Autodesk Fusion 360 part; units mm, degrees
note: some values were not read from the file. Set by a fixed rule: which sketch regions a step uses.
(part 2 of 3)
  line L909 (149.682, -103.079) -> (149.715, -103.248)
  line L910 (149.715, -103.248) -> (149.715, -103.421)
  line L911 (149.715, -103.421) -> (149.682, -103.59)
  line L912 (149.682, -103.59) -> (149.616, -103.749)
  line L913 (144.253, -97.1502) -> (144.186, -96.9907)
  line L914 (144.186, -96.9907) -> (144.153, -96.8214)
  line L915 (144.153, -96.8214) -> (144.153, -96.6488)
  line L916 (129.784, -101.74) -> (129.88, -101.597)
  line L917 (129.88, -101.597) -> (130.002, -101.475)
  line L918 (144.471, -96.0544) -> (144.614, -95.9585)
  line L919 (144.614, -95.9585) -> (144.774, -95.8925)
  line L920 (138.289, -101.26) -> (138.289, -101.432)
  line L921 (138.289, -101.432) -> (138.255, -101.601)
  line L922 (144.774, -95.8925) -> (144.943, -95.8588)
  line L923 (144.943, -95.8588) -> (145.115, -95.8588)
  line L924 (145.115, -95.8588) -> (145.285, -95.8925)
  line L925 (130.305, -101.313) -> (130.475, -101.279)
  line L926 (130.475, -101.279) -> (130.647, -101.279)
  line L927 (130.647, -101.279) -> (130.816, -101.313)
  line L928 (144.943, -97.6114) -> (144.774, -97.5777)
  line L929 (144.774, -97.5777) -> (144.614, -97.5117)
  line L930 (144.614, -97.5117) -> (144.471, -97.4158)
  line L931 (130.002, -101.475) -> (130.146, -101.379)
  line L932 (130.146, -101.379) -> (130.305, -101.313)
  line L933 (144.471, -97.4158) -> (144.348, -97.2937)
  line L934 (144.348, -97.2937) -> (144.253, -97.1502)
  line L935 (138.255, -101.601) -> (138.189, -101.76)
  line L936 (138.189, -101.76) -> (138.094, -101.904)
  line L937 (121.703, -93.6793) -> (122.022, -93.8112)
  line L938 (122.022, -93.8112) -> (122.309, -94.0027)
  line L939 (122.309, -94.0027) -> (122.552, -94.2464)
  line L940 (122.552, -94.2464) -> (122.744, -94.5331)
  line L941 (122.744, -94.5331) -> (122.876, -94.8515)
  line L942 (122.876, -94.8515) -> (122.943, -95.1896)
  line L943 (122.943, -95.1896) -> (122.943, -95.5344)
  line L944 (122.943, -95.5344) -> (122.876, -95.8725)
  line L945 (122.876, -95.8725) -> (122.744, -96.1909)
  line L946 (125.164, -115.998) -> (124.972, -115.711)
  line L947 (124.972, -115.711) -> (124.84, -115.392)
  line L948 (124.84, -115.392) -> (124.773, -115.054)
  line L949 (122.744, -96.1909) -> (122.552, -96.4776)
  line L950 (122.552, -96.4776) -> (122.309, -96.7213)
  line L951 (122.309, -96.7213) -> (122.022, -96.9128)
  line L952 (122.022, -96.9128) -> (121.703, -97.0447)
  line L953 (121.703, -97.0447) -> (121.365, -97.112)
  line L954 (137.669, -100.505) -> (137.828, -100.571)
  line L955 (137.828, -100.571) -> (137.972, -100.666)
  line L956 (121.365, -97.112) -> (121.021, -97.112)
  line L957 (121.021, -97.112) -> (120.683, -97.0447)
  line L958 (131.917, -103.479) -> (132.086, -103.512)
  line L959 (120.683, -97.0447) -> (120.364, -96.9128)
  line L960 (120.364, -96.9128) -> (120.077, -96.7213)
  line L961 (120.077, -96.7213) -> (119.834, -96.4776)
  line L962 (149.616, -102.919) -> (149.682, -103.079)
  line L963 (119.834, -96.4776) -> (119.642, -96.1909)
  line L964 (119.642, -96.1909) -> (119.51, -95.8725)
  line L965 (119.51, -95.8725) -> (119.443, -95.5344)
  line L966 (119.443, -95.5344) -> (119.443, -95.1896)
  line L967 (150.254, -115.751) -> (150.062, -116.038)
  line L968 (150.386, -115.432) -> (150.254, -115.751)
  line L969 (119.443, -95.1896) -> (119.51, -94.8515)
  line L970 (119.51, -94.8515) -> (119.642, -94.5331)
  line L971 (137.972, -100.666) -> (138.094, -100.788)
  line L972 (138.094, -100.788) -> (138.189, -100.932)
  line L973 (138.189, -100.932) -> (138.255, -101.091)
  line L974 (138.255, -101.091) -> (138.289, -101.26)
  line L975 (149.819, -116.281) -> (149.532, -116.473)
  line L976 (119.642, -94.5331) -> (119.834, -94.2464)
  line L977 (119.834, -94.2464) -> (120.077, -94.0027)
  line L978 (120.077, -94.0027) -> (120.364, -93.8112)
  line L979 (136.856, -91.8657) -> (136.734, -91.7438)
  line L980 (136.734, -91.7438) -> (136.639, -91.6005)
  line L981 (147.08, -77.3815) -> (147.212, -77.0631)
  line L982 (147.212, -77.0631) -> (147.404, -76.7764)
  line L983 (147.404, -76.7764) -> (147.647, -76.5327)
  line L984 (147.647, -76.5327) -> (147.934, -76.3412)
  line L985 (147.934, -76.3412) -> (148.253, -76.2093)
  line L986 (148.253, -76.2093) -> (148.591, -76.142)
  line L987 (147.08, -78.4025) -> (147.013, -78.0644)
  line L988 (147.013, -78.0644) -> (147.013, -77.7196)
  line L989 (147.013, -77.7196) -> (147.08, -77.3815)
  line L990 (147.344, -113.806) -> (147.587, -113.563)
  line L991 (147.587, -113.563) -> (147.874, -113.371)
  line L992 (147.647, -79.2513) -> (147.404, -79.0076)
  line L993 (147.404, -79.0076) -> (147.212, -78.7209)
  line L994 (147.212, -78.7209) -> (147.08, -78.4025)
  line L995 (124.892, -90.5982) -> (124.987, -90.7418)
  line L996 (124.987, -90.7418) -> (125.054, -90.9012)
  line L997 (125.054, -90.9012) -> (125.087, -91.0705)
  line L998 (133.703, -97.4272) -> (133.771, -97.591)
  line L999 (133.771, -97.591) -> (133.805, -97.7649)
  line L1000 (133.805, -97.7649) -> (133.805, -97.9421)
  line L1001 (129.88, -102.714) -> (129.784, -102.57)
  line L1002 (129.784, -102.57) -> (129.718, -102.411)
  line L1003 (135.385, -111.797) -> (135.226, -111.731)
  line L1004 (135.226, -111.731) -> (135.082, -111.635)
  line L1005 (135.082, -111.635) -> (134.96, -111.513)
  line L1006 (126.695, -113.132) -> (127.033, -113.199)
  line L1007 (135.896, -110.112) -> (136.056, -110.178)
  line L1008 (136.056, -110.178) -> (136.199, -110.274)
  line L1009 (126.351, -113.132) -> (126.695, -113.132)
  line L1010 (124.987, -91.5719) -> (124.892, -91.7155)
  line L1011 (124.892, -91.7155) -> (124.769, -91.8375)
  line L1012 (124.769, -91.8375) -> (124.626, -91.9334)
  line L1013 (124.84, -114.372) -> (124.972, -114.053)
  line L1014 (124.972, -114.053) -> (125.164, -113.766)
  line L1015 (125.164, -113.766) -> (125.407, -113.523)
  line L1016 (136.517, -111.041) -> (136.484, -111.21)
  line L1017 (136.484, -111.21) -> (136.417, -111.369)
  line L1018 (136.417, -111.369) -> (136.322, -111.513)
  line L1019 (134.765, -111.041) -> (134.765, -110.868)
  line L1020 (147.874, -113.371) -> (148.193, -113.239)
  line L1021 (148.193, -113.239) -> (148.531, -113.172)
  line L1022 (148.531, -113.172) -> (148.875, -113.172)
  line L1023 (148.875, -113.172) -> (149.213, -113.239)
  line L1024 (148.158, -103.893) -> (148.063, -103.749)
  line L1025 (126.495, -94.7136) -> (126.665, -94.68)
  line L1026 (126.665, -94.68) -> (126.837, -94.68)
  line L1027 (126.837, -94.68) -> (127.006, -94.7136)
  line L1028 (133.805, -96.2135) -> (132.005, -96.2135)
  line L1029 (129.718, -102.411) -> (129.685, -102.242)
  line L1030 (129.685, -102.242) -> (129.685, -102.069)
  line L1031 (129.685, -102.069) -> (129.718, -101.9)
  line L1032 (129.718, -101.9) -> (129.784, -101.74)
  line L1033 (148.753, -104.21) -> (148.584, -104.177)
  line L1034 (148.584, -104.177) -> (148.424, -104.111)
  line L1035 (148.424, -104.111) -> (148.281, -104.015)
  line L1036 (148.281, -104.015) -> (148.158, -103.893)
  line L1037 (136.322, -111.513) -> (136.199, -111.635)
  line L1038 (124.626, -91.9334) -> (124.466, -91.9995)
  line L1039 (124.466, -91.9995) -> (124.297, -92.0332)
  line L1040 (124.297, -92.0332) -> (124.125, -92.0332)
  line L1041 (136.199, -110.274) -> (136.322, -110.396)
  line L1042 (136.322, -110.396) -> (136.417, -110.539)
  line L1043 (148.925, -104.21) -> (148.753, -104.21)
  line L1044 (132.005, -96.2135) -> (132.005, -94.4135)
  line L1045 (132.005, -94.4135) -> (133.805, -94.4135)
  line L1046 (125.407, -113.523) -> (125.694, -113.331)
  line L1047 (125.694, -113.331) -> (126.013, -113.199)
  line L1048 (126.013, -113.199) -> (126.351, -113.132)
  line L1049 (130.305, -102.998) -> (130.146, -102.932)
  line L1050 (130.146, -102.932) -> (130.002, -102.836)
  line L1051 (130.002, -102.836) -> (129.88, -102.714)
  line L1052 (133.332, -97.0559) -> (133.479, -97.1544)
  line L1053 (133.479, -97.1544) -> (133.605, -97.2798)
  line L1054 (133.605, -97.2798) -> (133.703, -97.4272)
  line L1055 (137.159, -90.3446) -> (137.328, -90.311)
  line L1056 (137.328, -90.311) -> (137.5, -90.311)
  line L1057 (137.5, -90.311) -> (137.669, -90.3446)
  line L1058 (135.727, -111.83) -> (135.555, -111.83)
  line L1059 (135.555, -111.83) -> (135.385, -111.797)
  line L1060 (130.647, -103.032) -> (130.475, -103.032)
  line L1061 (130.475, -103.032) -> (130.305, -102.998)
  line L1062 (148.063, -103.749) -> (147.996, -103.59)
  line L1063 (147.996, -103.59) -> (147.963, -103.421)
  line L1064 (147.963, -103.421) -> (147.963, -103.248)
  line L1065 (147.963, -103.248) -> (147.996, -103.079)
  line L1066 (130.976, -102.932) -> (130.816, -102.998)
  line L1067 (130.816, -102.998) -> (130.647, -103.032)
  line L1068 (124.466, -90.3142) -> (124.626, -90.3803)
  line L1069 (124.626, -90.3803) -> (124.769, -90.4762)
  line L1070 (124.769, -90.4762) -> (124.892, -90.5982)
  line L1071 (146.953, -114.75) -> (147.02, -114.412)
  line L1072 (133.805, -94.4135) -> (133.805, -96.2135)
  line L1073 (144.015, -93.6928) -> (144.174, -93.7588)
  line L1074 (144.174, -93.7588) -> (144.318, -93.8547)
  line L1075 (133.805, -97.9421) -> (133.771, -98.116)
  line L1076 (133.771, -98.116) -> (133.703, -98.2798)
  line L1077 (133.703, -98.2798) -> (133.605, -98.4272)
  line L1078 (133.605, -98.4272) -> (133.479, -98.5526)
  line L1079 (136.417, -110.539) -> (136.484, -110.699)
  line L1080 (136.484, -110.699) -> (136.517, -110.868)
  line L1081 (136.517, -110.868) -> (136.517, -111.041)
  line L1082 (124.125, -92.0332) -> (123.955, -91.9995)
  line L1083 (123.955, -91.9995) -> (123.796, -91.9334)
  line L1084 (123.796, -91.9334) -> (123.652, -91.8375)
  line L1085 (124.773, -115.054) -> (124.773, -114.71)
  line L1086 (124.773, -114.71) -> (124.84, -114.372)
  line L1087 (133.479, -98.5526) -> (133.332, -98.6511)
  line L1088 (125.087, -91.0705) -> (125.087, -91.2432)
  line L1089 (125.087, -91.2432) -> (125.054, -91.4125)
  line L1090 (125.054, -91.4125) -> (124.987, -91.5719)
  line L1091 (126.07, -94.9977) -> (126.192, -94.8756)
  line L1092 (126.192, -94.8756) -> (126.336, -94.7797)
  line L1093 (126.336, -94.7797) -> (126.495, -94.7136)
  line L1094 (144.318, -93.8547) -> (144.44, -93.9768)
  line L1095 (144.44, -93.9768) -> (144.536, -94.1203)
  line L1096 (134.96, -111.513) -> (134.864, -111.369)
  line L1097 (134.864, -111.369) -> (134.798, -111.21)
  line L1098 (134.798, -111.21) -> (134.765, -111.041)
  line L1099 (136.199, -111.635) -> (136.056, -111.731)
  line L1100 (136.056, -111.731) -> (135.896, -111.797)
  line L1101 (135.896, -111.797) -> (135.727, -111.83)
  line L1102 (147.344, -116.038) -> (147.152, -115.751)
  line L1103 (147.587, -116.281) -> (147.344, -116.038)
  line L1104 (128.61, -100.514) -> (128.514, -100.371)
  line L1105 (128.514, -100.371) -> (128.448, -100.211)
  line L1106 (128.448, -100.211) -> (128.415, -100.042)
  line L1107 (128.415, -100.042) -> (128.415, -99.8694)
  line L1108 (128.415, -99.8694) -> (128.448, -99.7001)
  line L1109 (140.364, -88.7128) -> (140.205, -88.7789)
  line L1110 (140.205, -88.7789) -> (140.035, -88.8126)
  line L1111 (140.035, -88.8126) -> (139.863, -88.8126)
  line L1112 (146.693, -101.221) -> (146.693, -101.048)
  line L1113 (146.693, -101.048) -> (146.726, -100.879)
  line L1114 (146.726, -100.879) -> (146.793, -100.719)
  line L1115 (146.793, -100.719) -> (146.888, -100.576)
  line L1116 (147.02, -115.432) -> (146.953, -115.094)
  line L1117 (142.916, -94.791) -> (142.883, -94.6217)
  line L1118 (142.883, -94.6217) -> (142.883, -94.4491)
  line L1119 (142.883, -94.4491) -> (142.916, -94.2798)
  line L1120 (142.916, -94.2798) -> (142.983, -94.1203)
  line L1121 (144.015, -95.378) -> (143.845, -95.4117)
  line L1122 (143.845, -95.4117) -> (143.673, -95.4117)
  line L1123 (143.673, -95.4117) -> (143.504, -95.378)
  line L1124 (143.504, -95.378) -> (143.344, -95.3119)
  line L1125 (143.344, -95.3119) -> (143.201, -95.216)
  line L1126 (135.647, -97.2105) -> (135.497, -96.8476)
  line L1127 (135.497, -96.8476) -> (135.42, -96.4624)
  line L1128 (135.42, -96.4624) -> (135.42, -96.0696)
  line L1129 (135.42, -96.0696) -> (135.497, -95.6844)
  line L1130 (143.215, -109.175) -> (143.048, -108.926)
  line L1131 (143.048, -108.926) -> (142.934, -108.649)
  line L1132 (142.934, -108.649) -> (142.875, -108.354)
  line L1133 (135.727, -110.078) -> (135.896, -110.112)
  line L1134 (129.741, -106.287) -> (130.103, -106.437)
  line L1135 (130.103, -106.437) -> (130.43, -106.655)
  line L1136 (146.888, -100.576) -> (147.011, -100.454)
  line L1137 (147.011, -100.454) -> (147.154, -100.358)
  line L1138 (139.863, -87.06) -> (140.035, -87.06)
  line L1139 (140.035, -87.06) -> (140.205, -87.0936)
  line L1140 (122.868, -87.0782) -> (121.35, -87.9545)
  line L1141 (144.844, -106.739) -> (145.121, -106.853)
  line L1142 (145.121, -106.853) -> (145.37, -107.02)
  line L1143 (145.37, -107.02) -> (145.583, -107.233)
  line L1144 (144.318, -95.216) -> (144.174, -95.3119)
  line L1145 (144.174, -95.3119) -> (144.015, -95.378)
  line L1146 (139.391, -88.6169) -> (139.268, -88.4949)
  line L1147 (139.268, -88.4949) -> (139.173, -88.3513)
  line L1148 (139.173, -88.3513) -> (139.106, -88.1919)
  line L1149 (126.257, -93.7716) -> (126.162, -93.9152)
  line L1150 (126.162, -93.9152) -> (126.039, -94.0372)
  line L1151 (126.039, -94.0372) -> (125.896, -94.1331)
  line L1152 (125.896, -94.1331) -> (125.736, -94.1992)
  line L1153 (134.765, -110.868) -> (134.798, -110.699)
  line L1154 (134.798, -110.699) -> (134.864, -110.539)
  line L1155 (134.864, -110.539) -> (134.96, -110.396)
  line L1156 (135.647, -95.3215) -> (135.865, -94.995)
  line L1157 (135.865, -94.995) -> (136.143, -94.7172)
  line L1158 (136.143, -94.7172) -> (136.47, -94.499)
  line L1159 (128.963, -110.198) -> (128.577, -110.121)
  line L1160 (128.577, -110.121) -> (128.215, -109.971)
  line L1161 (128.215, -109.971) -> (127.888, -109.753)
  line L1162 (143.201, -95.216) -> (143.078, -95.094)
  line L1163 (143.078, -95.094) -> (142.983, -94.9505)
  line L1164 (142.983, -94.9505) -> (142.916, -94.791)
  line L1165 (145.583, -109.175) -> (145.37, -109.388)
  line L1166 (145.37, -109.388) -> (145.121, -109.555)
  line L1167 (128.963, -106.21) -> (129.355, -106.21)
  line L1168 (129.355, -106.21) -> (129.741, -106.287)
  line L1169 (131.076, -108.786) -> (130.926, -109.148)
  line L1170 (130.926, -109.148) -> (130.708, -109.475)
  line L1171 (130.708, -109.475) -> (130.43, -109.753)
  line L1172 (129.035, -100.798) -> (128.876, -100.732)
  line L1173 (139.106, -87.6807) -> (139.173, -87.5212)
  line L1174 (139.173, -87.5212) -> (139.268, -87.3777)
  line L1175 (139.268, -87.3777) -> (139.391, -87.2556)
  line L1176 (128.876, -100.732) -> (128.732, -100.636)
  line L1177 (128.732, -100.636) -> (128.61, -100.514)
  line L1178 (130.43, -106.655) -> (130.708, -106.933)
  line L1179 (136.47, -98.033) -> (136.143, -97.8148)
  line L1180 (136.143, -97.8148) -> (135.865, -97.537)
  line L1181 (135.865, -97.537) -> (135.647, -97.2105)
  line L1182 (139.863, -88.8126) -> (139.694, -88.7789)
  line L1183 (139.694, -88.7789) -> (139.534, -88.7128)
  line L1184 (139.534, -88.7128) -> (139.391, -88.6169)
  line L1185 (127.888, -106.655) -> (128.215, -106.437)
  line L1186 (128.215, -106.437) -> (128.577, -106.287)
  line L1187 (128.577, -106.287) -> (128.963, -106.21)
  line L1188 (130.43, -109.753) -> (130.103, -109.971)
  line L1189 (130.103, -109.971) -> (129.741, -110.121)
  line L1190 (129.741, -110.121) -> (129.355, -110.198)
  line L1191 (125.395, -94.2329) -> (125.225, -94.1992)
  line L1192 (125.225, -94.1992) -> (125.066, -94.1331)
  line L1193 (127.61, -106.933) -> (127.888, -106.655)
  line L1194 (140.726, -88.3513) -> (140.63, -88.4949)
  line L1195 (140.63, -88.4949) -> (140.508, -88.6169)
  line L1196 (140.508, -88.6169) -> (140.364, -88.7128)
  line L1197 (130.708, -106.933) -> (130.926, -107.26)
  line L1198 (130.926, -107.26) -> (131.076, -107.622)
  line L1199 (131.076, -107.622) -> (131.153, -108.008)
  line L1200 (127.888, -109.753) -> (127.61, -109.475)
  line L1201 (127.61, -109.475) -> (127.392, -109.148)
  line L1202 (145.121, -109.555) -> (144.844, -109.669)
  line L1203 (144.844, -109.669) -> (144.549, -109.728)
  line L1204 (144.549, -109.728) -> (144.249, -109.728)
  line L1205 (127.392, -109.148) -> (127.242, -108.786)
  line L1206 (127.242, -108.786) -> (127.165, -108.4)
  line L1207 (127.165, -108.4) -> (127.165, -108.008)
  line L1208 (135.497, -95.6844) -> (135.647, -95.3215)
  line L1209 (147.152, -115.751) -> (147.02, -115.432)
  line L1210 (148.193, -116.605) -> (147.874, -116.473)
  line L1211 (146.953, -115.094) -> (146.953, -114.75)
  line L1212 (149.213, -116.605) -> (148.875, -116.672)
  line L1213 (142.875, -108.354) -> (142.875, -108.054)
  line L1214 (142.875, -108.054) -> (142.934, -107.759)
  line L1215 (131.15, -103.796) -> (131.272, -103.674)
  line L1216 (142.934, -107.759) -> (143.048, -107.482)
  line L1217 (143.048, -107.482) -> (143.215, -107.233)
  line L1218 (143.215, -107.233) -> (143.428, -107.02)
  line L1219 (145.923, -108.354) -> (145.864, -108.649)
  line L1220 (145.864, -108.649) -> (145.75, -108.926)
  line L1221 (145.75, -108.926) -> (145.583, -109.175)
  line L1222 (145.923, -108.054) -> (145.923, -108.354)
  line L1223 (127.165, -108.008) -> (127.242, -107.622)
  line L1224 (127.242, -107.622) -> (127.392, -107.26)
  line L1225 (127.392, -107.26) -> (127.61, -106.933)
  line L1226 (139.106, -88.1919) -> (139.073, -88.0226)
  line L1227 (139.073, -88.0226) -> (139.073, -87.85)
  line L1228 (139.073, -87.85) -> (139.106, -87.6807)
  line L1229 (147.874, -116.473) -> (147.587, -116.281)
  line L1230 (148.875, -116.672) -> (148.531, -116.672)
  line L1231 (143.428, -109.388) -> (143.215, -109.175)
  line L1232 (144.635, -94.6217) -> (144.602, -94.791)
  line L1233 (144.602, -94.791) -> (144.536, -94.9505)
  line L1234 (144.536, -94.9505) -> (144.44, -95.094)
  line L1235 (144.44, -95.094) -> (144.318, -95.216)
  line L1236 (136.47, -94.499) -> (136.832, -94.3487)
  line L1237 (136.832, -94.3487) -> (137.218, -94.2721)
  line L1238 (137.218, -94.2721) -> (137.61, -94.2721)
  line L1239 (145.583, -107.233) -> (145.75, -107.482)
  line L1240 (145.75, -107.482) -> (145.864, -107.759)
  line L1241 (145.864, -107.759) -> (145.923, -108.054)
  line L1242 (125.736, -94.1992) -> (125.567, -94.2329)
  line L1243 (125.567, -94.2329) -> (125.395, -94.2329)
  line L1244 (150.062, -116.038) -> (149.819, -116.281)
  line L1245 (147.02, -114.412) -> (147.152, -114.093)
  line L1246 (147.152, -114.093) -> (147.344, -113.806)
  line L1247 (135.226, -110.178) -> (135.385, -110.112)
  line L1248 (135.385, -110.112) -> (135.555, -110.078)
  line L1249 (135.555, -110.078) -> (135.727, -110.078)
  line L1250 (146.793, -101.55) -> (146.726, -101.39)
  line L1251 (146.726, -101.39) -> (146.693, -101.221)
  line L1252 (139.391, -87.2556) -> (139.534, -87.1597)
  line L1253 (139.534, -87.1597) -> (139.694, -87.0936)
  line L1254 (139.694, -87.0936) -> (139.863, -87.06)
  line L1255 (125.066, -94.1331) -> (124.922, -94.0372)
  line L1256 (124.922, -94.0372) -> (124.8, -93.9152)
  line L1257 (124.8, -93.9152) -> (124.704, -93.7716)
  line L1258 (124.704, -93.7716) -> (124.638, -93.6122)
  line L1259 (129.355, -110.198) -> (128.963, -110.198)
  line L1260 (144.249, -109.728) -> (143.954, -109.669)
  line L1261 (143.954, -109.669) -> (143.677, -109.555)
  line L1262 (143.677, -109.555) -> (143.428, -109.388)
  line L1263 (134.96, -110.396) -> (135.082, -110.274)
  line L1264 (135.082, -110.274) -> (135.226, -110.178)
  line L1265 (131.153, -108.008) -> (131.153, -108.4)
  line L1266 (131.153, -108.4) -> (131.076, -108.786)
  line L1267 (135.052, -109.313) -> (134.929, -109.435)
  line L1268 (131.404, -102.411) -> (131.337, -102.57)
  line L1269 (131.337, -102.57) -> (131.242, -102.714)
  line L1270 (131.242, -102.714) -> (131.119, -102.836)
  line L1271 (131.119, -102.836) -> (130.976, -102.932)
  line L1272 (147.825, -101.977) -> (147.655, -102.011)
  line L1273 (147.655, -102.011) -> (147.483, -102.011)
  line L1274 (134.188, -78.5788) -> (134.311, -78.4568)
  line L1275 (134.311, -78.4568) -> (134.454, -78.3609)
  line L1276 (134.454, -78.3609) -> (134.614, -78.2948)
  line L1277 (125.908, -95.3007) -> (125.974, -95.1412)
  line L1278 (125.974, -95.1412) -> (126.07, -94.9977)
  line L1279 (128.276, -98.5986) -> (128.107, -98.6323)
  line L1280 (128.107, -98.6323) -> (127.935, -98.6323)
  line L1281 (127.935, -98.6323) -> (127.765, -98.5986)
  line L1282 (133.495, -108.841) -> (133.495, -108.668)
  line L1283 (143.428, -107.02) -> (143.677, -106.853)
  line L1284 (143.677, -106.853) -> (143.954, -106.739)
  line L1285 (143.954, -106.739) -> (144.249, -106.68)
  line L1286 (126.07, -96.1149) -> (125.974, -95.9714)
  line L1287 (125.974, -95.9714) -> (125.908, -95.8119)
  line L1288 (125.395, -92.4803) -> (125.567, -92.4803)
  line L1289 (125.567, -92.4803) -> (125.736, -92.5139)
  line L1290 (134.929, -109.435) -> (134.786, -109.531)
  line L1291 (134.786, -109.531) -> (134.626, -109.597)
  line L1292 (134.626, -109.597) -> (134.457, -109.631)
  line L1293 (129.972, -99.3971) -> (130.067, -99.5406)
  line L1294 (130.067, -99.5406) -> (130.134, -99.7001)
  line L1295 (130.134, -99.7001) -> (130.167, -99.8694)
  line L1296 (130.167, -99.8694) -> (130.167, -100.042)
  line L1297 (130.167, -100.042) -> (130.134, -100.211)
  line L1298 (147.825, -100.292) -> (147.984, -100.358)
  line L1299 (147.984, -100.358) -> (148.128, -100.454)
  line L1300 (130.134, -100.211) -> (130.067, -100.371)
  line L1301 (144.549, -106.68) -> (144.844, -106.739)
  line L1302 (134.626, -107.912) -> (134.786, -107.978)
  line L1303 (134.786, -107.978) -> (134.929, -108.074)
  line L1304 (148.346, -100.719) -> (148.412, -100.879)
  line L1305 (148.412, -100.879) -> (148.445, -101.048)
  line L1306 (148.445, -101.048) -> (148.445, -101.221)
  line L1307 (128.579, -97.0753) -> (128.702, -97.1974)
  line L1308 (128.702, -97.1974) -> (128.797, -97.3409)
  line L1309 (128.797, -97.3409) -> (128.864, -97.5004)
  line L1310 (150.122, -76.7764) -> (150.314, -77.0631)
  line L1311 (150.314, -77.0631) -> (150.446, -77.3815)
  line L1312 (150.446, -77.3815) -> (150.513, -77.7196)
  line L1313 (127.61, -85.599) -> (127.392, -85.2725)
  line L1314 (127.392, -85.2725) -> (127.242, -84.9096)
  line L1315 (127.242, -84.9096) -> (127.165, -84.5244)
  line L1316 (129.849, -100.636) -> (129.706, -100.732)
  line L1317 (129.706, -100.732) -> (129.546, -100.798)
  line L1318 (129.546, -100.798) -> (129.377, -100.832)
  line L1319 (129.377, -100.832) -> (129.205, -100.832)
  line L1320 (129.205, -100.832) -> (129.035, -100.798)
  line L1321 (149.273, -76.2093) -> (149.592, -76.3412)
  line L1322 (149.592, -76.3412) -> (149.879, -76.5327)
  line L1323 (149.879, -76.5327) -> (150.122, -76.7764)
  line L1324 (127.432, -96.1149) -> (127.309, -96.2369)
  line L1325 (127.309, -96.2369) -> (127.166, -96.3328)
  line L1326 (133.993, -79.0511) -> (134.026, -78.8818)
  line L1327 (134.026, -78.8818) -> (134.093, -78.7224)
  line L1328 (134.093, -78.7224) -> (134.188, -78.5788)
  line L1329 (142.745, -91.4931) -> (142.904, -91.5591)
  line L1330 (142.904, -91.5591) -> (143.048, -91.655)
  line L1331 (143.048, -91.655) -> (143.17, -91.7771)
  line L1332 (143.17, -91.7771) -> (143.266, -91.9206)
  line L1333 (149.592, -79.4428) -> (149.273, -79.5747)
  line L1334 (149.273, -79.5747) -> (148.935, -79.642)
  line L1335 (148.935, -79.642) -> (148.591, -79.642)
  line L1336 (148.128, -100.454) -> (148.25, -100.576)
  line L1337 (148.25, -100.576) -> (148.346, -100.719)
  line L1338 (127.627, -95.6426) -> (127.594, -95.8119)
  line L1339 (127.594, -95.8119) -> (127.527, -95.9714)
  line L1340 (127.527, -95.9714) -> (127.432, -96.1149)
  line L1341 (126.665, -96.4326) -> (126.495, -96.3989)
  line L1342 (126.495, -96.3989) -> (126.336, -96.3328)
  line L1343 (126.336, -96.3328) -> (126.192, -96.2369)
  line L1344 (126.192, -96.2369) -> (126.07, -96.1149)
  line L1345 (134.614, -78.2948) -> (134.783, -78.2611)
  line L1346 (134.783, -78.2611) -> (134.955, -78.2611)
  line L1347 (134.955, -78.2611) -> (135.125, -78.2948)
  line L1348 (143.266, -91.9206) -> (143.332, -92.0801)
  line L1349 (143.332, -92.0801) -> (143.365, -92.2494)
  line L1350 (135.247, -108.841) -> (135.214, -109.01)
  line L1351 (135.214, -109.01) -> (135.147, -109.17)
  line L1352 (135.147, -109.17) -> (135.052, -109.313)
  line L1353 (125.908, -95.8119) -> (125.875, -95.6426)
  line L1354 (125.875, -95.6426) -> (125.875, -95.47)
  line L1355 (125.875, -95.47) -> (125.908, -95.3007)
  line L1356 (131.242, -101.597) -> (131.337, -101.74)
  line L1357 (131.337, -101.74) -> (131.404, -101.9)
  line L1358 (131.404, -101.9) -> (131.437, -102.069)
  line L1359 (131.437, -102.069) -> (131.437, -102.242)
  line L1360 (134.929, -108.074) -> (135.052, -108.196)
  line L1361 (135.052, -108.196) -> (135.147, -108.339)
  line L1362 (130.708, -85.599) -> (130.43, -85.8768)
  line L1363 (130.43, -85.8768) -> (130.103, -86.095)
  line L1364 (130.103, -86.095) -> (129.741, -86.2453)
  line L1365 (128.864, -98.0116) -> (128.797, -98.1711)
  line L1366 (128.797, -98.1711) -> (128.702, -98.3146)
  line L1367 (128.702, -98.3146) -> (128.579, -98.4366)
  line L1368 (128.579, -98.4366) -> (128.436, -98.5325)
  line L1369 (133.495, -108.668) -> (133.528, -108.499)
  line L1370 (133.528, -108.499) -> (133.594, -108.339)
  line L1371 (133.594, -108.339) -> (133.69, -108.196)
  line L1372 (127.765, -98.5986) -> (127.606, -98.5325)
  line L1373 (127.606, -98.5325) -> (127.462, -98.4366)
  line L1374 (127.462, -98.4366) -> (127.34, -98.3146)
  line L1375 (150.513, -77.7196) -> (150.513, -78.0644)
  line L1376 (150.513, -78.0644) -> (150.446, -78.4025)
  line L1377 (150.446, -78.4025) -> (150.314, -78.7209)
  line L1378 (133.69, -109.313) -> (133.594, -109.17)
  line L1379 (133.594, -109.17) -> (133.528, -109.01)
  line L1380 (133.528, -109.01) -> (133.495, -108.841)
  line L1381 (128.436, -98.5325) -> (128.276, -98.5986)
  line L1382 (148.445, -101.221) -> (148.412, -101.39)
  line L1383 (148.412, -101.39) -> (148.346, -101.55)
  line L1384 (134.115, -109.597) -> (133.956, -109.531)
  line L1385 (133.956, -109.531) -> (133.812, -109.435)
  line L1386 (133.812, -109.435) -> (133.69, -109.313)
  line L1387 (150.314, -78.7209) -> (150.122, -79.0076)
  line L1388 (150.122, -79.0076) -> (149.879, -79.2513)
  line L1389 (149.879, -79.2513) -> (149.592, -79.4428)
  line L1390 (127.166, -96.3328) -> (127.006, -96.3989)
  line L1391 (127.006, -96.3989) -> (126.837, -96.4326)
  line L1392 (126.837, -96.4326) -> (126.665, -96.4326)
  line L1393 (129.741, -86.2453) -> (129.355, -86.3219)
  line L1394 (129.355, -86.3219) -> (128.963, -86.3219)
  line L1395 (128.963, -86.3219) -> (128.577, -86.2453)
  line L1396 (127.165, -84.5244) -> (127.165, -84.1316)
  line L1397 (127.165, -84.1316) -> (127.242, -83.7464)
  line L1398 (127.242, -83.7464) -> (127.392, -83.3835)
  line L1399 (130.067, -100.371) -> (129.972, -100.514)
  line L1400 (129.972, -100.514) -> (129.849, -100.636)
  line L1401 (143.365, -92.2494) -> (143.365, -92.422)
  line L1402 (143.365, -92.422) -> (143.332, -92.5913)
  line L1403 (147.483, -102.011) -> (147.314, -101.977)
  line L1404 (147.314, -101.977) -> (147.154, -101.911)
  line L1405 (128.577, -86.2453) -> (128.215, -86.095)
  line L1406 (128.215, -86.095) -> (127.888, -85.8768)
  line L1407 (127.888, -85.8768) -> (127.61, -85.599)
  line L1408 (128.436, -96.9794) -> (128.579, -97.0753)
  line L1409 (131.119, -101.475) -> (131.242, -101.597)
  line L1410 (143.332, -92.5913) -> (143.266, -92.7508)
  line L1411 (143.266, -92.7508) -> (143.17, -92.8943)
  line L1412 (143.17, -92.8943) -> (143.048, -93.0163)
  line L1413 (143.048, -93.0163) -> (142.904, -93.1122)
  line L1414 (128.864, -97.5004) -> (128.897, -97.6697)
  line L1415 (128.897, -97.6697) -> (128.897, -97.8423)
  line L1416 (128.897, -97.8423) -> (128.864, -98.0116)
  line L1417 (134.093, -79.5525) -> (134.026, -79.3931)
  line L1418 (134.026, -79.3931) -> (133.993, -79.2238)
  line L1419 (133.993, -79.2238) -> (133.993, -79.0511)
  line L1420 (134.457, -109.631) -> (134.285, -109.631)
  line L1421 (134.285, -109.631) -> (134.115, -109.597)
  line L1422 (148.346, -101.55) -> (148.25, -101.693)
  line L1423 (148.25, -101.693) -> (148.128, -101.815)
  line L1424 (148.128, -101.815) -> (147.984, -101.911)
  line L1425 (147.984, -101.911) -> (147.825, -101.977)
  line L1426 (144.249, -106.68) -> (144.549, -106.68)
  line L1427 (135.147, -108.339) -> (135.214, -108.499)
  line L1428 (135.214, -108.499) -> (135.247, -108.668)
  line L1429 (135.247, -108.668) -> (135.247, -108.841)
  line L1430 (131.437, -102.242) -> (131.404, -102.411)
  line L1431 (149.819, -113.563) -> (150.062, -113.806)
  line L1432 (149.532, -113.371) -> (149.819, -113.563)
  line L1433 (149.213, -113.239) -> (149.532, -113.371)
  line L1434 (127.033, -113.199) -> (127.352, -113.331)
  line L1435 (127.352, -113.331) -> (127.639, -113.523)
  line L1436 (127.639, -113.523) -> (127.882, -113.766)
  line L1437 (150.254, -114.093) -> (150.386, -114.412)
  line L1438 (150.062, -113.806) -> (150.254, -114.093)
  line L1439 (144.449, -105.321) -> (144.321, -105.268)
  line L1440 (144.321, -105.268) -> (144.207, -105.192)
  line L1441 (144.207, -105.192) -> (144.109, -105.094)
  line L1442 (131.917, -105.231) -> (131.745, -105.231)
  line L1443 (131.272, -103.674) -> (131.416, -103.579)
  line L1444 (131.416, -103.579) -> (131.575, -103.512)
  line L1445 (131.575, -103.512) -> (131.745, -103.479)
  line L1446 (131.745, -103.479) -> (131.917, -103.479)
  line L1447 (141.931, -91.655) -> (142.074, -91.5591)
  line L1448 (142.074, -91.5591) -> (142.234, -91.4931)
  line L1449 (136.539, -101.26) -> (136.573, -101.091)
  line L1450 (136.573, -101.091) -> (136.639, -100.932)
  line L1451 (136.639, -100.932) -> (136.734, -100.788)
  line L1452 (136.639, -91.6005) -> (136.573, -91.4412)
  line L1453 (136.573, -91.4412) -> (136.539, -91.2722)
  line L1454 (136.539, -91.2722) -> (136.539, -91.0998)
  line L1455 (132.512, -103.796) -> (132.607, -103.94)
  line L1456 (132.607, -103.94) -> (132.674, -104.099)
  line L1457 (132.674, -104.099) -> (132.707, -104.269)
  line L1458 (138.963, -94.995) -> (139.181, -95.3215)
  line L1459 (139.181, -95.3215) -> (139.331, -95.6844)
  line L1460 (139.331, -95.6844) -> (139.408, -96.0696)
  line L1461 (146.858, -99.6155) -> (146.714, -99.7114)
  line L1462 (146.714, -99.7114) -> (146.555, -99.7774)
  line L1463 (146.555, -99.7774) -> (146.385, -99.8111)
  line L1464 (146.385, -99.8111) -> (146.213, -99.8111)
  line L1465 (146.213, -99.8111) -> (146.044, -99.7774)
  line L1466 (131.272, -105.036) -> (131.15, -104.914)
  line L1467 (131.15, -104.914) -> (131.054, -104.77)
  line L1468 (127.166, -94.7797) -> (127.309, -94.8756)
  line L1469 (127.309, -94.8756) -> (127.432, -94.9977)
  line L1470 (127.432, -94.9977) -> (127.527, -95.1412)
  line L1471 (127.527, -95.1412) -> (127.594, -95.3007)
  line L1472 (144.321, -104.028) -> (144.449, -103.975)
  line L1473 (144.449, -103.975) -> (144.584, -103.948)
  line L1474 (144.584, -103.948) -> (144.722, -103.948)
  line L1475 (144.722, -105.348) -> (144.584, -105.348)
  line L1476 (144.584, -105.348) -> (144.449, -105.321)
  line L1477 (144.722, -103.948) -> (144.857, -103.975)
  line L1478 (132.086, -103.512) -> (132.246, -103.579)
  line L1479 (132.246, -103.579) -> (132.389, -103.674)
  line L1480 (131.745, -105.231) -> (131.575, -105.198)
  line L1481 (131.575, -105.198) -> (131.416, -105.132)
  line L1482 (131.416, -105.132) -> (131.272, -105.036)
  line L1483 (137.669, -102.187) -> (137.5, -102.221)
  line L1484 (137.5, -102.221) -> (137.328, -102.221)
  line L1485 (144.109, -105.094) -> (144.033, -104.98)
  line L1486 (144.033, -104.98) -> (143.98, -104.852)
  line L1487 (143.98, -104.852) -> (143.953, -104.717)
  line L1488 (132.707, -104.269) -> (132.707, -104.441)
  line L1489 (132.707, -104.441) -> (132.674, -104.611)
  line L1490 (138.094, -90.6282) -> (138.189, -90.7715)
  line L1491 (138.189, -90.7715) -> (138.255, -90.9308)
  line L1492 (127.145, -97.6697) -> (127.178, -97.5004)
  line L1493 (127.882, -113.766) -> (128.074, -114.053)
  line L1494 (128.074, -114.053) -> (128.206, -114.372)
  line L1495 (136.539, -91.0998) -> (136.573, -90.9308)
  line L1496 (136.573, -90.9308) -> (136.639, -90.7715)
  line L1497 (136.639, -90.7715) -> (136.734, -90.6282)
  line L1498 (146.044, -99.7774) -> (145.884, -99.7114)
  line L1499 (130.955, -104.269) -> (130.988, -104.099)
  line L1500 (130.988, -104.099) -> (131.054, -103.94)
  line L1501 (131.054, -103.94) -> (131.15, -103.796)
  line L1502 (141.613, -92.2494) -> (141.646, -92.0801)
  line L1503 (141.646, -92.0801) -> (141.713, -91.9206)
  line L1504 (141.713, -91.9206) -> (141.808, -91.7771)
  line L1505 (141.808, -91.7771) -> (141.931, -91.655)
  line L1506 (132.389, -103.674) -> (132.512, -103.796)
  line L1507 (142.575, -91.4594) -> (142.745, -91.4931)
  line L1508 (137.669, -90.3446) -> (137.828, -90.4106)
  line L1509 (137.828, -90.4106) -> (137.972, -90.5063)
  line L1510 (137.972, -90.5063) -> (138.094, -90.6282)
  line L1511 (132.674, -104.611) -> (132.607, -104.77)
  line L1512 (132.607, -104.77) -> (132.512, -104.914)
  line L1513 (132.512, -104.914) -> (132.389, -105.036)
  line L1514 (138.094, -101.904) -> (137.972, -102.026)
  line L1515 (137.972, -102.026) -> (137.828, -102.121)
  line L1516 (137.828, -102.121) -> (137.669, -102.187)
  line L1517 (145.884, -99.7114) -> (145.741, -99.6155)
  line L1518 (145.741, -99.6155) -> (145.618, -99.4934)
  line L1519 (141.646, -92.5913) -> (141.613, -92.422)
  line L1520 (141.613, -92.422) -> (141.613, -92.2494)
  line L1521 (144.109, -104.202) -> (144.207, -104.104)
  line L1522 (144.207, -104.104) -> (144.321, -104.028)
  line L1523 (145.618, -99.4934) -> (145.523, -99.3499)
  line L1524 (145.523, -99.3499) -> (145.456, -99.1904)
  line L1525 (145.456, -99.1904) -> (145.423, -99.0211)
  line L1526 (145.423, -99.0211) -> (145.423, -98.8485)
  line L1527 (145.423, -98.8485) -> (145.456, -98.6792)
  line L1528 (136.734, -101.904) -> (136.639, -101.76)
  line L1529 (136.639, -101.76) -> (136.573, -101.601)
  line L1530 (136.734, -90.6282) -> (136.856, -90.5063)
  line L1531 (136.856, -90.5063) -> (137, -90.4106)
  line L1532 (137, -90.4106) -> (137.159, -90.3446)
  line L1533 (143.953, -104.717) -> (143.953, -104.579)
  line L1534 (142.234, -91.4931) -> (142.403, -91.4594)
  line L1535 (142.403, -91.4594) -> (142.575, -91.4594)
  line L1536 (147.076, -99.3499) -> (146.98, -99.4934)
  line L1537 (146.98, -99.4934) -> (146.858, -99.6155)
  line L1538 (138.685, -94.7172) -> (138.963, -94.995)
  line L1539 (127.34, -98.3146) -> (127.244, -98.1711)
  line L1540 (127.244, -98.1711) -> (127.178, -98.0116)
  line L1541 (127.178, -98.0116) -> (127.145, -97.8423)
  line L1542 (127.145, -97.8423) -> (127.145, -97.6697)
  line L1543 (127.935, -96.8797) -> (128.107, -96.8797)
  line L1544 (128.107, -96.8797) -> (128.276, -96.9133)
  line L1545 (137.996, -94.3487) -> (138.358, -94.499)
  line L1546 (138.358, -94.499) -> (138.685, -94.7172)
  line L1547 (128.206, -114.372) -> (128.273, -114.71)
  line L1548 (128.273, -114.71) -> (128.273, -115.054)
  line L1549 (128.273, -115.054) -> (128.206, -115.392)
  line L1550 (145.741, -98.2541) -> (145.884, -98.1582)
  line L1551 (145.884, -98.1582) -> (146.044, -98.0922)
  line L1552 (146.044, -98.0922) -> (146.213, -98.0585)
  line L1553 (146.213, -98.0585) -> (146.385, -98.0585)
  line L1554 (146.385, -98.0585) -> (146.555, -98.0922)
  line L1555 (145.456, -98.6792) -> (145.523, -98.5197)
  line L1556 (147.142, -99.1904) -> (147.076, -99.3499)
  line L1557 (141.808, -92.8943) -> (141.713, -92.7508)
  line L1558 (141.713, -92.7508) -> (141.646, -92.5913)
  line L1559 (136.573, -101.601) -> (136.539, -101.432)
  line L1560 (136.539, -101.432) -> (136.539, -101.26)
  line L1561 (131.054, -104.77) -> (130.988, -104.611)
  line L1562 (130.988, -104.611) -> (130.955, -104.441)
  line L1563 (130.955, -104.441) -> (130.955, -104.269)
  line L1564 (143.953, -104.579) -> (143.98, -104.444)
  line L1565 (143.98, -104.444) -> (144.033, -104.316)
  line L1566 (144.033, -104.316) -> (144.109, -104.202)
  line L1567 (137.328, -102.221) -> (137.159, -102.187)
  line L1568 (137.159, -102.187) -> (137, -102.121)
  line L1569 (137, -102.121) -> (136.856, -102.026)
  line L1570 (136.856, -102.026) -> (136.734, -101.904)
  line L1571 (127.594, -95.3007) -> (127.627, -95.47)
  line L1572 (127.627, -95.47) -> (127.627, -95.6426)
  line L1573 (127.178, -97.5004) -> (127.244, -97.3409)
  line L1574 (127.244, -97.3409) -> (127.34, -97.1974)
  line L1575 (127.34, -97.1974) -> (127.462, -97.0753)
  line L1576 (145.523, -98.5197) -> (145.618, -98.3762)
  line L1577 (145.618, -98.3762) -> (145.741, -98.2541)
  line L1578 (132.389, -105.036) -> (132.246, -105.132)
  line L1579 (132.246, -105.132) -> (132.086, -105.198)
  line L1580 (132.086, -105.198) -> (131.917, -105.231)
  line L1581 (127.462, -97.0753) -> (127.606, -96.9794)
  line L1582 (127.606, -96.9794) -> (127.765, -96.9133)
  line L1583 (127.765, -96.9133) -> (127.935, -96.8797)
  line L1584 (138.935, -84.8939) -> (139.094, -84.96)
  line L1585 (139.094, -84.96) -> (139.238, -85.0559)
  line L1586 (139.238, -85.0559) -> (139.36, -85.178)
  line L1587 (139.555, -85.6503) -> (139.555, -85.8229)
  line L1588 (139.555, -85.8229) -> (139.522, -85.9922)
  line L1589 (139.522, -85.9922) -> (139.456, -86.1516)
  line L1590 (139.36, -85.178) -> (139.456, -85.3215)
  line L1591 (139.456, -85.3215) -> (139.522, -85.481)
  line L1592 (139.522, -85.481) -> (139.555, -85.6503)
  line L1593 (121.021, -93.612) -> (121.365, -93.612)
  line L1594 (121.365, -93.612) -> (121.703, -93.6793)
  line L1595 (127.006, -94.7136) -> (127.166, -94.7797)
  line L1596 (124.605, -93.2703) -> (124.638, -93.101)
  line L1597 (124.638, -93.101) -> (124.704, -92.9415)
  line L1598 (124.704, -92.9415) -> (124.8, -92.798)
  line L1599 (124.8, -92.798) -> (124.922, -92.6759)
  line L1600 (124.922, -92.6759) -> (125.066, -92.58)
  line L1601 (132.817, -98.7535) -> (132.643, -98.7189)
  line L1602 (132.643, -98.7189) -> (132.479, -98.6511)
  line L1603 (132.479, -98.6511) -> (132.332, -98.5526)
  line L1604 (132.332, -98.5526) -> (132.206, -98.4272)
  line L1605 (132.206, -98.4272) -> (132.108, -98.2798)
  line L1606 (132.108, -98.2798) -> (132.04, -98.116)
  line L1607 (132.04, -98.116) -> (132.005, -97.9421)
  line L1608 (125.066, -92.58) -> (125.225, -92.5139)
  line L1609 (125.225, -92.5139) -> (125.395, -92.4803)
  line L1610 (121.35, -87.9545) -> (120.474, -86.4367)
  line L1611 (120.474, -86.4367) -> (121.992, -85.5604)
  line L1612 (121.992, -85.5604) -> (122.868, -87.0782)
  line L1613 (133.332, -98.6511) -> (133.168, -98.7189)
  line L1614 (133.168, -98.7189) -> (132.994, -98.7535)
  line L1615 (132.994, -98.7535) -> (132.817, -98.7535)
  line L1616 (147.483, -100.258) -> (147.655, -100.258)
  line L1617 (147.655, -100.258) -> (147.825, -100.292)
  line L1618 (129.546, -99.1131) -> (129.706, -99.1791)
  line L1619 (129.355, -82.3341) -> (129.741, -82.4107)
  line L1620 (144.844, -82.8626) -> (145.121, -82.9774)
  line L1621 (145.121, -82.9774) -> (145.37, -83.1442)
  line L1622 (145.37, -83.1442) -> (145.583, -83.3565)
  line L1623 (145.583, -83.3565) -> (145.75, -83.6061)
  line L1624 (145.75, -83.6061) -> (145.864, -83.8835)
  line L1625 (129.706, -99.1791) -> (129.849, -99.275)
  line L1626 (129.849, -99.275) -> (129.972, -99.3971)
  line L1627 (133.168, -96.9881) -> (133.332, -97.0559)
  line L1628 (126.357, -93.4429) -> (126.324, -93.6122)
  line L1629 (126.324, -93.6122) -> (126.257, -93.7716)
  line L1630 (128.732, -99.275) -> (128.876, -99.1791)
  line L1631 (128.876, -99.1791) -> (129.035, -99.1131)
  line L1632 (129.035, -99.1131) -> (129.205, -99.0794)
  line L1633 (129.205, -99.0794) -> (129.377, -99.0794)
  line L1634 (129.377, -99.0794) -> (129.546, -99.1131)
  line L1635 (126.162, -92.798) -> (126.257, -92.9415)
  line L1636 (126.257, -92.9415) -> (126.324, -93.101)
  line L1637 (126.324, -93.101) -> (126.357, -93.2703)
  line L1638 (126.357, -93.2703) -> (126.357, -93.4429)
  line L1639 (146.555, -98.0922) -> (146.714, -98.1582)
  line L1640 (128.215, -82.561) -> (128.577, -82.4107)
  line L1641 (128.577, -82.4107) -> (128.963, -82.3341)
  line L1642 (128.963, -82.3341) -> (129.355, -82.3341)
  line L1643 (145.864, -83.8835) -> (145.923, -84.1779)
  line L1644 (145.923, -84.1779) -> (145.923, -84.4781)
  line L1645 (145.923, -84.4781) -> (145.864, -84.7725)
  line L1646 (127.392, -83.3835) -> (127.61, -83.057)
  line L1647 (127.61, -83.057) -> (127.888, -82.7792)
  line L1648 (127.888, -82.7792) -> (128.215, -82.561)
  line L1649 (137.61, -98.2599) -> (137.218, -98.2599)
  line L1650 (137.218, -98.2599) -> (136.832, -98.1833)
  line L1651 (136.832, -98.1833) -> (136.47, -98.033)
  line L1652 (128.514, -99.5406) -> (128.61, -99.3971)
  line L1653 (128.61, -99.3971) -> (128.732, -99.275)
  line L1654 (147.996, -103.079) -> (148.063, -102.919)
  line L1655 (148.584, -102.492) -> (148.753, -102.458)
  line L1656 (139.181, -97.2105) -> (138.963, -97.537)
  line L1657 (138.963, -97.537) -> (138.685, -97.8148)
  line L1658 (138.685, -97.8148) -> (138.358, -98.033)
  line L1659 (138.358, -98.033) -> (137.996, -98.1833)
  line L1660 (142.983, -94.1203) -> (143.078, -93.9768)
  line L1661 (143.078, -93.9768) -> (143.201, -93.8547)
  line L1662 (137.996, -98.1833) -> (137.61, -98.2599)
  line L1663 (141.996, -89.7209) -> (142.062, -89.8804)
  line L1664 (142.062, -89.8804) -> (142.095, -90.0497)
  line L1665 (142.095, -90.0497) -> (142.095, -90.2223)
  line L1666 (148.063, -102.919) -> (148.158, -102.776)
  line L1667 (148.158, -102.776) -> (148.281, -102.654)
  line L1668 (148.281, -102.654) -> (148.424, -102.558)
  line L1669 (148.424, -102.558) -> (148.584, -102.492)
  line L1670 (150.386, -114.412) -> (150.453, -114.75)
  line L1671 (141.634, -89.3594) -> (141.778, -89.4553)
  line L1672 (141.778, -89.4553) -> (141.9, -89.5774)
  line L1673 (141.9, -89.5774) -> (141.996, -89.7209)
  line L1674 (147.154, -101.911) -> (147.011, -101.815)
  line L1675 (147.011, -101.815) -> (146.888, -101.693)
  line L1676 (146.888, -101.693) -> (146.793, -101.55)
  line L1677 (148.591, -76.142) -> (148.935, -76.142)
  line L1678 (148.935, -76.142) -> (149.273, -76.2093)
  line L1679 (139.408, -96.0696) -> (139.408, -96.4624)
  line L1680 (139.408, -96.4624) -> (139.331, -96.8476)
  line L1681 (139.331, -96.8476) -> (139.181, -97.2105)
  line L1682 (119.443, -95.362) -> (122.943, -95.362) construction
  line L1683 (147.013, -77.892) -> (150.513, -77.892) construction
  line L1684 (146.953, -114.922) -> (150.453, -114.922) construction
  line L1685 (128.273, -114.882) -> (124.773, -114.882) construction
  point P0 (150.034, -75.927)
  point P1 (150.738, -76.6319)
  point P2 (150.718, -116.274)
  point P3 (150.123, -116.867)
  point P4 (125.094, -116.865)
  point P5 (124.562, -116.338)
  point P6 (124.562, -97.7901)
  point P7 (124.078, -97.307)
  point P8 (119.76, -97.307)
  point P9 (119.228, -96.7802)
  point P10 (132.254, -75.9171)
  point P11 (119.226, -80.7196)
  point P12 (122.943, -95.362)
  point P13 (119.443, -95.362)
  point P14 (121.193, -95.362)
  point P15 (147.013, -77.892)
  point P16 (150.513, -77.892)
  point P17 (148.763, -77.892)
  point P18 (146.953, -114.922)
  point P19 (150.453, -114.922)
  point P20 (148.703, -114.922)
  point P21 (128.273, -114.882)
  point P22 (124.773, -114.882)
  point P23 (126.523, -114.882)
  constraint coincident P0 L228.end
  constraint coincident P1 L54.start
  constraint coincident P2 L7.end
  constraint coincident P3 L38.start
  constraint coincident P4 L2.start
  constraint coincident P5 L21.end
  constraint coincident P6 L123.start
  constraint coincident P7 L359.start
  constraint coincident P8 L319.start
  constraint coincident P9 L239.start
  constraint coincident P10 L103.start
  constraint coincident P11 L222.start
  constraint midpoint L943 P12
  constraint midpoint L966 P13
  constraint coincident P13 L1682.start
  constraint coincident P12 L1682.end
  constraint perpendicular L943 L1682
  constraint midpoint L1682 P14
  constraint midpoint L988 P15
  constraint midpoint L1375 P16
  constraint coincident P15 L1683.start
  constraint coincident P16 L1683.end
  constraint perpendicular L1375 L1683
  constraint midpoint L1683 P17
  constraint midpoint L1211 P18
  constraint midpoint L559 P19
  constraint coincident P18 L1684.start
  constraint coincident P19 L1684.end
  constraint perpendicular L559 L1684
  constraint midpoint L1684 P20
  constraint midpoint L1548 P21
  constraint midpoint L1085 P22
  constraint coincident P21 L1685.start
  constraint coincident P22 L1685.end
  constraint perpendicular L1085 L1685
  constraint midpoint L1685 P23